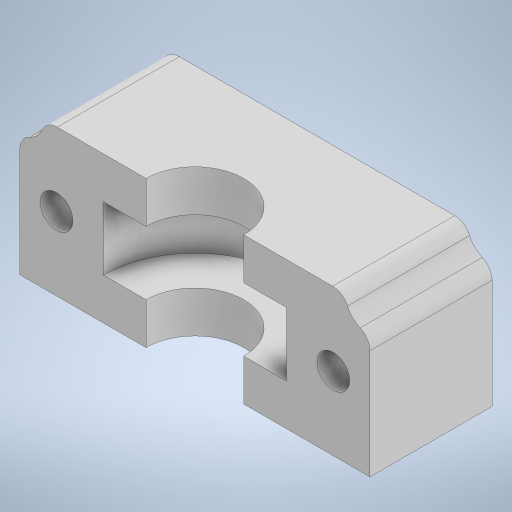
# Autodesk Inventor part: bearing_holder_v3
Saved by Autodesk Inventor 2024 (Build 280153000, 153)
## iProperties
Created: 2024-02-02
Part Number: bearing_holder_v3
Material: Generic
Document SubType Name: Modeling
Designer: Pintu
Density: 1 g/cm^3
Appearance: Default
Author: Pintu
Autodesk Inventor part; units mm, degrees
ref_plane "YZ Plane" through (0, 0, 0) normal (1, 0, 0) x (0, 1, 0)
ref_plane "XZ Plane" through (0, 0, 0) normal (0, 1, 0) x (-1, 0, 0)
sketch "Sketch1" plane through (0, 0, 0) normal (0, 0, 1) x (1, 0, 0)
  line L0 (-21.5, 9) -> (21.5, 9)
  line L1 (21.5, 9) -> (21.5, -9)
  line L2 (21.5, -9) -> (-21.5, -9)
  line L3 (-21.5, -9) -> (-21.5, 9)
  line L4 (-21.5, 9) -> (21.5, -9) construction
  line L5 (21.5, 9) -> (-21.5, -9) construction
  point P0 (0, 0)
  dimension "d0" = 43
  dimension "d1" = 18
  constraints: 12 end point, 2 midpoint, 2 parallel, 1 horizontal, 1 perpendicular
  measures "d0" distance of L1.end L2.end
  measures "d1" distance of L0.end L1.end
extrude "Extrusion1" add sketch "Sketch1" along normal blind 15
ref_plane "Work Plane1" through (-21.5, 0, 0) normal (0, 1, 0) x (1, 0, 0)
sketch "Sketch2" plane through (-21.5, 0, 0) normal (0, 1, 0) x (1, 0, 0)
  line L0 (0, -15) -> (43, -15) projected
  circle A0 centre (21.5, -15) radius 11.25
  point P0 (21.5, 0)
  dimension "d4" = 22.5
  constraints: 1 centre point, 1 midpoint
  measures "d4" diameter of A0
extrude "Extrusion2" cut sketch "Sketch2" along normal mid plane 7.8
sketch "Sketch3" plane through (-21.5, 0, 0) normal (0, 1, 0) x (1, 0, 0)
  line L0 (10.25, -15) -> (32.75, -15) projected
  arc A0 (32.75, -15) -> (10.25, -15) centre (21.5, -15) ccw projected
  circle A1 centre (21.5, -15) radius 6
  point P0 (21.5, 0)
  dimension "d7" = 12
  constraints: 1 centre point, 1 coincident
  measures "d7" diameter of A1
extrude "Extrusion3" cut sketch "Sketch3" along normal mid plane 26.75 contours A1 L0 | L0 A1
sketch "Sketch4" plane through (0, 0, 0) normal (0, 0, -1) x (-1, 0, 0)
  line L0 (21.5, 9) -> (21.5, -9) projected
  line L1 (21.5, -9) -> (-21.5, -9) projected
  point P0 (0, 0)
  point P1 (17, 0)
  dimension "d10" = 4.5
  dimension "d11" = 9
  measures "d10" distance from line of L0 point (17, 0)
  measures "d11" distance from line of L1 point (17, 0)
hole "Hole1" at (-17, 0, 0) direction (0, 0, 1) diameter 4 depth 25 tip angle 118 counterbore diameter 7 counterbore depth 4
sketch "Sketch5" plane through (0, 0, 0) normal (0, 0, -1) x (-1, 0, 0)
  line L0 (-21.5, -9) -> (-21.5, 9) projected
  line L1 (21.5, -9) -> (-21.5, -9) projected
  point P0 (0, 0)
  point P1 (-17, 0)
  dimension "sideOff" = 4.5
  dimension "d20" = 9
  measures "sideOff" distance from line of L0 point (-17, 0)
  measures "d20" distance from line of L1 point (-17, 0)
hole "Hole2" at (17, 0, 0) direction (0, 0, 1) diameter 4 depth 25 tip angle 118 counterbore diameter 7 counterbore depth 4
fillet "Fillet1" radius 3 2 edges at (21.5, 9, 7.5) (-21.5, 9, 7.5) inverted yes
fillet "Fillet2" radius 2 4 edges at (21.5, 6, 7.5) (18.5, 9, 7.5) (-18.5, 9, 7.5) (-21.5, 6, 7.5)
equation "\"d10\" = sideOff"
body "Solid1"
